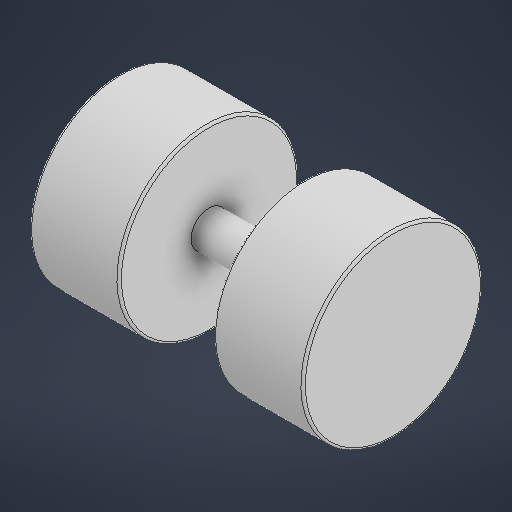
# Autodesk Inventor part: součást 2
Saved by Autodesk Inventor 2025.1 (Build 291241000, 241)
## iProperties
Created: 2025-04-28
Part Number: součást 2
Material: Všeobecné
Document SubType Name: Modeling
Designer: Dominik Petříček
Density: 1 g/cm^3
Appearance: Výchozí
Author: Dominik Petříček
Autodesk Inventor part; units mm, degrees
ref_plane "YZ Plane" through (0, 0, 0) normal (1, 0, 0) x (0, 1, 0)
ref_plane "XZ Plane" through (0, 0, 0) normal (0, 1, 0) x (-1, 0, 0)
ref_plane "XY Plane" through (0, 0, 0) normal (0, 0, 1) x (1, 0, 0)
sketch "Náčrt1" plane through (0, 0, 0) normal (0, 0, 1) x (1, 0, 0)
  line L0 (0, 0) -> (0, -19.5)
  line L1 (0.5, -20) -> (19.5, -20)
  line L2 (20, -19.5) -> (20, 0)
  line L3 (20, 0) -> (20, -4)
  line L4 (20, -4) -> (41, -4)
  line L5 (41, -4) -> (41, -19.5)
  line L6 (41.5, -20) -> (60.5, -20)
  line L7 (61, -19.5) -> (61, 0)
  line L8 (61, 0) -> (0, 0)
  arc A0 (41, -19.5) -> (41.5, -20) centre (41.5, -19.5) ccw
  arc A1 (60.5, -20) -> (61, -19.5) centre (60.5, -19.5) ccw
  arc A2 (0, -19.5) -> (0.5, -20) centre (0.5, -19.5) ccw
  arc A3 (19.5, -20) -> (20, -19.5) centre (19.5, -19.5) ccw
  point P0 (0, -20)
  point P1 (20, -20)
  point P2 (41, -20)
  point P3 (61, -20)
  dimension "d0" = 20
  dimension "d1" = 20
  dimension "d2" = 20
  dimension "d3" = 4
  dimension "d4" = 21
  dimension "d5" = 90
  dimension "d6" = 20
  dimension "d7" = 90
  dimension "d9" = 0.5
  dimension "d10" = 0.5
  constraints: 18 end point, 11 point on line, 8 point on circle, 8 tangent, 4 centre point, 4 perpendicular, 2 equal radius, 1 vertical
  measures "d0" distance of L0.start point (0, -20)
  measures "d1" distance of point (0, -20) point (20, -20)
  measures "d2" distance of point (20, -20) L2.end
  measures "d3" distance of L2.end L3.end
  measures "d4" distance of L3.end L4.end
  measures "d5" angle of L4 L5
  measures "d6" distance of point (41, -20) point (61, -20)
  measures "d7" angle of L7 L6
  measures "d9" radius of A0
  measures "d10" radius of A2
revolve "Rotace1" add sketch "Náčrt1" angle 360 about axis through (61, 0, 0) along (-1, 0, 0)
